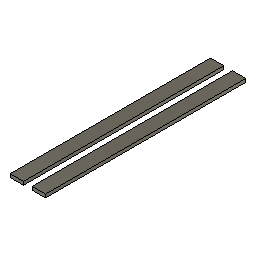
cnc (Autodesk Fusion 360 design; units mm, degrees)
Autodesk Fusion 360 part; units mm, degrees
sketch "Sketch1" plane through (0, 0, 0) normal (0, 0, 1) x (1, 0, 0)
  line L0 (-100, 75) -> (200, 75)
  line L1 (200, 75) -> (200, -225)
  line L2 (200, -225) -> (-100, -225)
  line L3 (-100, -225) -> (-100, 75)
  dimension "d1" = 300
  dimension "d2" = 300
  constraint perpendicular L0 L1
  constraint parallel L0 L2
  constraint parallel L1 L3
  constraint horizontal L0
  measures "d1" distance of L0.start L0.end
  measures "d2" distance of L0.start L2.end
extrude "Extrude1" add sketch "Sketch1" along normal blind 5 makes body 1
sketch "Sketch2" plane through (0, 0, 5) normal (0, 0, 1) x (-1, 0, 0)
  line L0 (100, 225) -> (-200, 225)
  line L1 (-200, 225) -> (-200, -75)
  line L2 (-200, -75) -> (100, -75)
  line L3 (100, -75) -> (100, 225)
  line L4 (100, -75) -> (80, -75)
  line L5 (80, -75) -> (80, 225)
  line L6 (80, 225) -> (100, 225)
  line L7 (100, 225) -> (100, -75)
  dimension "d5" = 20
  dimension "d6" = 300
  constraint perpendicular L4 L5
  constraint parallel L4 L6
  constraint parallel L5 L7
  constraint perpendicular L3 L4
  constraint coincident L2.end L3.start
  measures "d5" distance of L2.end L4.end
  measures "d6" distance of L2.end L0.start
extrude "Extrude2" add sketch "Sketch2" along normal blind 5 contours L0 L2 L3 L4 L5 L6 L7 bodies 1
sketch "Sketch3" plane through (0, 0, 5) normal (0, 0, 1) x (-1, 0, 0)
  line L0 (80, -75) -> (80, 225)
  line L1 (80, 225) -> (-200, 225)
  line L2 (-200, 225) -> (-200, -75)
  line L3 (-200, -75) -> (80, -75)
  line L4 (67.0832, -75) -> (47.0832, -75)
  line L5 (47.0832, -75) -> (47.0832, 225)
  line L6 (47.0832, 225) -> (67.0832, 225)
  line L7 (67.0832, 225) -> (67.0832, -75)
  dimension "d9" = 20
  dimension "d10" = 300
  constraint perpendicular L4 L5
  constraint parallel L4 L6
  constraint parallel L5 L7
  constraint parallel L3 L4
  constraint coincident L3 L4.start
  measures "d9" distance of L4.start L4.end
  measures "d10" distance of L4.start L6.end
extrude "Extrude3" add sketch "Sketch3" along normal blind 5 contours L1 L3 L4 L5 L6 L7 bodies 1
extrude "Extrude4" cut 1 faces at (0, -25, 0) along direction (0, 0, 1) blind 5 on bodies 1 bodies 1 makes body 2 at (-60.4166, -125, 5)
